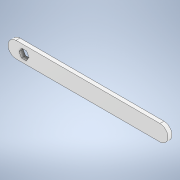
# Autodesk Inventor part: armForTurningControlWheel
Saved by Autodesk Inventor 2020.2 (Build 242310000, 310)
## iProperties
Created: 2020-02-01
Part Number: armForTurningControlWheel
Material: PBT Plastic
Document SubType Name: Modeling
Designer: robst
Density: 1.31 g/cm^3
Appearance: Snow
Author: robst
Autodesk Inventor part; units mm, degrees
ref_plane "YZ Plane" through (0, 0, 0) normal (1, 0, 0) x (0, 1, 0)
ref_plane "XZ Plane" through (0, 0, 0) normal (0, 1, 0) x (-1, 0, 0)
ref_plane "XY Plane" through (0, 0, 0) normal (0, 0, 1) x (1, 0, 0)
sketch "Sketch1" plane through (0, 0, 0) normal (0, 0, 1) x (1, 0, 0)
  line L0 (-114.3, -12.7) -> (114.3, -12.7)
  line L1 (114.3, 12.7) -> (-114.3, 12.7)
  line L2 (-127, -12.7) -> (127, 12.7) construction
  line L3 (127, -12.7) -> (-127, 12.7) construction
  line L4 (-93.6811, -0.2452) -> (-97.6405, -7.1032)
  line L5 (-97.6405, -7.1032) -> (-105.5595, -7.1032)
  line L6 (-105.5595, -7.1032) -> (-109.5189, -0.2452)
  line L7 (-109.5189, -0.2452) -> (-105.5595, 6.6128)
  line L8 (-105.5595, 6.6128) -> (-97.6405, 6.6128)
  line L9 (-97.6405, 6.6128) -> (-93.6811, -0.2452)
  arc A0 (-114.3, 12.7) -> (-114.3, -12.7) centre (-114.3, 0) ccw
  arc A1 (114.3, -12.7) -> (114.3, 12.7) centre (114.3, 0) ccw
  point P0 (0, 0)
  point P1 (-101.6, -0.2452)
  dimension "d0" = 254
  dimension "d1" = 25.4
  dimension "d2" = 13.716
  dimension "d14" = 25.4
  constraints: 20 end point, 4 point on circle, 3 tangent, 2 centre point, 2 horizontal, 2 midpoint, 1 parallel, 13 other
  measures "d0" distance of L2.end L3.end
  measures "d1" distance of L3.end L2.start
  measures "d2" distance between parallel lines of L5 L8
  measures "d14" diameter of A1
extrude "Extrusion4" add sketch "Sketch1" along normal mid plane 6.35
body "Solid2"
